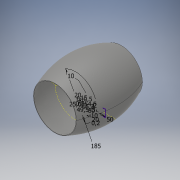
# Autodesk Inventor part: Form
Saved by Autodesk Inventor 2018.3 (Build 223284000, 284)
## iProperties
Created: 2018-07-22
Part Number: Form
Material: Generisch
Document SubType Name: Modeling
Designer: JochenAlt
Density: 1 g/cm^3
Appearance: Textur - grau
Author: JochenAlt
Autodesk Inventor part; units mm, degrees
ref_plane "YZ Plane" through (0, 0, 0) normal (1, 0, 0) x (0, 1, 0)
ref_plane "XZ Plane" through (0, 0, 0) normal (0, 1, 0) x (-1, 0, 0)
ref_plane "XY Plane" through (0, 0, 0) normal (0, 0, 1) x (1, 0, 0)
sketch "Skizze3" plane through (0, 0, 0) normal (0, 0, 1) x (1, 0, 0)
  line L0 (0, 279.6242) -> (0, -256.3919) construction
  line L1 (-139.5878, 0) -> (207.5271, 0) construction
  line L2 (92, 200) -> (90, 200)
  circle A0 centre (0, 0) radius 90 construction
  circle A1 centre (0, -90) radius 89.8182 construction
  line L3 (92, -90) -> (94, -90)
  line L4 (92, -90) -> (155.9392, 64.9092) construction
  line L5 (155.9392, 64.9092) -> (90, 200) construction
  spline S0 degree 2 poles (92, -90) (155.9392, 64.9092) (90, 200) knots 1 1 1 2 2 2
  line L6 (92, 200) -> (157.9392, 64.9092) construction
  line L7 (157.9392, 64.9092) -> (94, -90) construction
  spline S1 degree 2 poles (92, 200) (157.9392, 64.9092) (94, -90) knots 1 1 1 2 2 2
  line L8 (155.9392, 64.9092) -> (157.9392, 64.9092) construction
  line L9 (155.9392, 64.9092) -> (157.9392, 64.9092) construction
  point P0 (90, 149.8145)
  dimension "d7" = 200
  dimension "d11" = 2
  dimension "d12" = 92
  dimension "d13" = 180
  dimension "d14" = 90
  dimension "d15" = 90
  dimension "d18" = 2
  dimension "d19" = 2
  constraints: 8 end point, 4 horizontal, 3 coincident, 2 centre point, 2 point on line, 1 parallel, 6 other
  measures "d7" distance between parallel lines of L1 L2
  measures "d11" distance of L2.start L2.end
  measures "d12" distance from line of L0 L3.start
  measures "d13" diameter of A0
  measures "d14" distance of A1.centre point (0, 0)
  measures "d15" distance from line of L0 L2.end
  measures "d18" distance of L3.end L3.start
  measures "d19" distance of L8.start L8.end
revolve "Umdrehung1" add sketch "Skizze3" angle 360 about axis through (0, 0, 0) along (0, -1, 0)
sketch "Skizze6" plane through (0, 0, 0) normal (1, 0, 0) x (0, 1, 0)
  line L0 (-40, 0) -> (240, 0) construction
  line L1 (0, 126) -> (0, -126) construction
  line L2 (179, 25) -> (179, -25)
  line L3 (184, 25) -> (179, 25)
  line L4 (179, -25) -> (184, -25)
  line L5 (184, -25) -> (184, 25)
  line L6 (200, 90) -> (200, -90) projected
  point P0 (0, 0)
  point P1 (200, 0)
  dimension "d35" = 50
  dimension "d49" = 16
  dimension "d51" = 5
  constraints: 8 end point, 2 vertical, 1 horizontal, 1 parallel, 1 other
  measures "d35" distance of L2.start L2.end
  measures "d49" distance between parallel lines of L6 L5
  measures "d51" distance of L2.end L4.end
extrude "Extrusion4" add sketch "Skizze6" along normal up to next separate body
sketch "Skizze7" plane through (0, 0, 0) normal (0, 1, 0) x (-1, 0, 0)
  arc A0 (-91.7745, 11.5625) -> (-91.7745, -11.5625) centre (0, 0) ccw
  circle A1 centre (-80, 0) radius 7.6
  line L0 (-78.75, -9.9216) -> (-91.7745, -11.5625)
  line L1 (-78.75, 9.9216) -> (-91.7745, 11.5625)
  line L2 (-92, 0) -> (-125.4773, 0) construction
  arc A2 (-78.75, -9.9216) -> (-78.75, 9.9216) centre (-80, 0) ccw
  circle A3 centre (-80, 0) radius 6.6
  line L3 (-91.7745, -11.5625) -> (-130, -16.3785)
  line L4 (-91.7745, 11.5625) -> (-130, 16.3785)
  line L5 (-130, -16.3785) -> (-130, 16.3785)
  line L6 (-84.7731, 8.6646) -> (-84.5231, 10.6489) construction
  circle A4 centre (0, 0) radius 90 construction
  line L7 (0, 0) -> (-44.9, -77.7691) construction
  line L8 (0, 0) -> (-44.9, 77.7691) construction
  arc A5 (-44.9, 77.7691) -> (-44.9, -77.7691) centre (0, 0) ccw
  arc A6 (-34.9, 60.4486) -> (-34.9, -60.4486) centre (0, 0) ccw
  line L9 (-44.9, -77.7691) -> (-34.9, -60.4486)
  line L10 (-44.9, 77.7691) -> (-34.9, 60.4486)
  line L11 (-73.0798, -13.4093) -> (-28.2175, 7.5103) construction
  line L12 (-28.2175, 7.5103) -> (-23.9914, -1.5528) construction
  line L13 (-23.9914, -1.5528) -> (-68.8536, -22.4724) construction
  line L14 (-68.8536, -22.4724) -> (-73.0798, -13.4093) construction
  circle A7 centre (-73.0798, -13.4093) radius 1.5
  circle A8 centre (-68.8536, -22.4724) radius 1.5
  circle A9 centre (-23.9914, -1.5528) radius 1.5
  circle A10 centre (-28.2175, 7.5103) radius 1.5
  line L15 (-26.1045, 2.9788) -> (-70.9667, -17.9408) construction
  circle A11 centre (-39.6991, -3.3605) radius 1.8416 construction
  line L16 (-77.4586, -9.9343) -> (-28.0649, 13.0984) construction
  line L17 (-28.0649, 13.0984) -> (-19.6125, -5.0278) construction
  line L18 (-19.6125, -5.0278) -> (-69.0063, -28.0605) construction
  line L19 (-69.0063, -28.0605) -> (-77.4586, -9.9343) construction
  line L20 (-52.7618, 1.5821) -> (-44.3094, -16.5441) construction
  line L21 (-70.8879, -6.8703) -> (-62.4355, -24.9965) construction
  line L22 (-34.6356, 10.0344) -> (-26.1832, -8.0917) construction
  line L23 (-174, 0) -> (134, 0) construction
  line L24 (-34.3938, 10.6989) -> (-21.3136, -17.3515)
  line L25 (-30.112, 18.0801) -> (-15.5806, -13.0825)
  line L26 (-71.9053, -5.8716) -> (-60.6811, -29.942)
  line L27 (-77.8164, -9.7587) -> (-67.8386, -31.1561)
  line L28 (-34.3938, 10.6989) -> (-73.346, -7.4648)
  point P0 (-69.1582, 8.7131)
  point P1 (-94, 0)
  point P2 (-90, 0)
  point P3 (-77.6568, -9.7216)
  point P4 (-87.7427, 11.0545)
  dimension "d32" = 185
  dimension "d40" = 15.2
  dimension "d50" = 80
  dimension "d52" = 10
  dimension "d53" = 1
  dimension "d56" = 50
  dimension "d67" = 2
  dimension "d71" = 0.2
  dimension "d72" = 20
  dimension "d90" = 49.5
  dimension "d91" = 10
  dimension "d92" = 3
  dimension "d93" = 15
  dimension "d94" = 54.5
  dimension "d95" = 20
  dimension "d96" = 40
  dimension "d97" = 25
  dimension "d98" = 0.5
  dimension "d99" = 7
  dimension "d100" = 0.5
  constraints: 54 end point, 12 point on circle, 12 point on line, 11 centre point, 9 coincident, 7 parallel, 5 perpendicular, 4 midpoint, 3 equal radius, 2 collinear, 2 tangent, 1 horizontal alignment, 1 vertical, 6 other
  measures "d32" diameter of A0
  measures "d40" diameter of A1
  measures "d50" distance of A1.centre point (0, 0)
  measures "d52" radius of A2
  measures "d53" radial gap between concentric circles of A3 A1
  measures "d56" distance from line of L5 A1.centre
  measures "d67" distance of L6.start L6.end
  measures "d72" radial gap between concentric circles of A5 A6
  measures "d90" distance of L12.end L13.end
  measures "d91" distance of L13.end L11.start
  measures "d92" diameter of A7
  measures "d93" distance from line of L12 A11.centre
  measures "d94" distance of L16.start L16.end
  measures "d95" distance of L16.end L17.end
  measures "d96" distance between parallel lines of L21 L22
  measures "d97" angle of L23 L15
  measures "d98" distance between parallel lines of L24 L22
  measures "d99" distance between parallel lines of L25 L24
  measures "d100" distance between parallel lines of L28 L16
extrude "Extrusion5" cut sketch "Skizze7" along normal through all both and the other way through all contours L1 A5 L0 A0 | A0 L3 L5 L4 | L1 A2 L0 A5 keep common part bodies 2
extrude "Extrusion8" add sketch "Skizze7" along normal blind 1 from surface at 179 contours A1 bodies 2
extrude "Extrusion9" add sketch "Skizze7" along normal blind 1 from surface at 179 contours A1 bodies 2
pattern_circular "Runde Anordnung2" count 3 over 360 about axis through (0, -10, 0) along (0, 1, 0) bodies 2
combine bodies "Kombinieren2" operation type add bodies to combine 2 1
extrude "Extrusion10" add sketch "Skizze7" against normal blind 1 from surface at 200 separate body contours A5 L10 A6 L28 L26 A2 L1 | L1 A2 L0 A5 | L0 A2 L28 L26 A6 L9 A5 | L26 L28 A2 | L28 A6 L26 | A1 | A7 | A8
extrude "Extrusion11" add sketch "Skizze7" against normal blind 4 from surface at 199 contours A5 L10 A6 L28 L26 A2 L1 | L1 A2 L0 A5 | L0 A2 L28 L26 A6 L9 A5 | L26 L28 A2 | L28 A6 L26 | A7 | A8 bodies 3
pattern_circular "Runde Anordnung3" count 3 over 360 about axis through (0, -10, 0) along (0, 1, 0) of "Extrusion10", "Extrusion11" bodies 3
equation "\"d14\" = 0.5 * d13"
equation "\"d18\" = d17"
equation "\"d16\" = d11"
equation "\"d17\" = d16"
